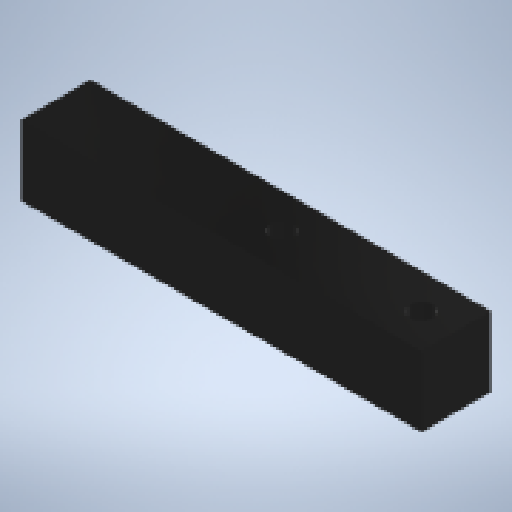
# Autodesk Inventor part: Tope X
Saved by Autodesk Inventor 2023 (Build 270158000, 158)
## iProperties
Created: 2024-01-18
Part Number: Tope X
Material: Polypropylene
Document SubType Name: Modeling
Designer: juanp
Density: 0.899 g/cm^3
Appearance: Smooth - Black
Author: juanp
Autodesk Inventor part; units mm, degrees
ref_plane "YZ Plane" through (0, 0, 0) normal (1, 0, 0) x (0, 1, 0)
ref_plane "XZ Plane" through (0, 0, 0) normal (0, 1, 0) x (-1, 0, 0)
ref_plane "XY Plane" through (0, 0, 0) normal (0, 0, 1) x (1, 0, 0)
sketch "Sketch1" plane through (0, 0, 0) normal (0, 1, 0) x (-1, 0, 0)
  line L0 (85, 5) -> (0, 5)
  line L1 (0, 5) -> (0, -5)
  line L2 (0, -5) -> (85, -5)
  line L3 (85, -5) -> (85, 5)
  line L4 (25, 0) -> (5, 0) construction
  circle A0 centre (25, 0) radius 1.65
  circle A1 centre (5, 0) radius 1.65
  point P0 (0, 0)
  point P1 (0, 0)
  dimension "d0" = 10
  dimension "d1" = 20
  dimension "d2" = 3.3
  dimension "d3" = 5
  dimension "d6" = 85
  constraints: 10 end point, 3 coincident, 2 centre point, 2 horizontal, 2 parallel, 1 equal radius, 1 midpoint, 1 perpendicular, 1 point on line
  measures "d0" distance between parallel lines of L2 L0
  measures "d1" distance of L4.start L4.end
  measures "d2" diameter of A0
  measures "d3" distance from line of L4.end L1
  measures "d6" distance of L0.start L0.end
extrude "Extrusion1" add sketch "Sketch1" along normal blind 10
body "Solid1"
